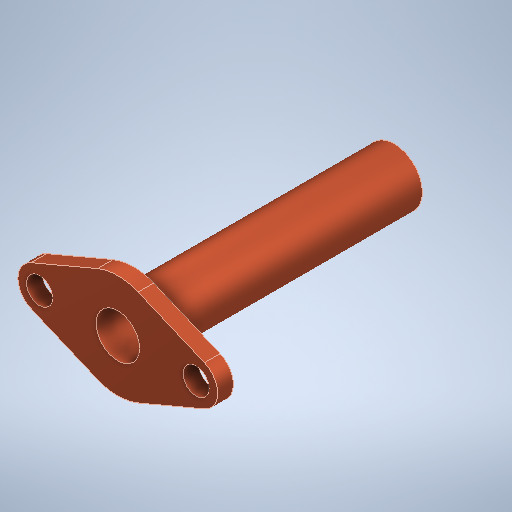
# Autodesk Inventor part: 36 - Inlet Outlet Steam Pipe
Saved by Autodesk Inventor 2025.2 (Build 292293000, 293)
## iProperties
Created: 2025-07-30
Part Number: 36 - Inlet Outlet Steam Pipe
Material: Copper
Document SubType Name: Modeling
Designer: bless
Density: 8.94 g/cm^3
Appearance: Copper - Satin
Author: bless
Autodesk Inventor part; units mm, degrees
ref_plane "YZ Plane" through (0, 0, 0) normal (1, 0, 0) x (0, 1, 0)
ref_plane "XZ Plane" through (0, 0, 0) normal (0, 1, 0) x (-1, 0, 0)
ref_plane "XY Plane" through (0, 0, 0) normal (0, 0, 1) x (1, 0, 0)
sketch "Sketch1" plane through (0, 0, 0) normal (0, 0, 1) x (1, 0, 0)
  circle A0 centre (0, 0) radius 2.5
  circle A1 centre (9, 0) radius 1.5
  circle A2 centre (-9, 0) radius 1.5
  circle A3 centre (-9, 0) radius 2.5
  circle A4 centre (9, 0) radius 2.5
  circle A5 centre (0, 0) radius 6
  line L0 (-9.9722, 2.3032) -> (-2.3333, 5.5277)
  line L1 (9.9722, 2.3032) -> (2.3333, 5.5277)
  line L2 (-9.9722, -2.3032) -> (-2.3333, -5.5277)
  line L3 (9.9722, -2.3032) -> (2.3333, -5.5277)
  dimension "d0" = 5
  dimension "d1" = 3
  dimension "d2" = 3
  dimension "d4" = 9
  dimension "d5" = 9
  dimension "d6" = 5
  dimension "d7" = 5
  dimension "d8" = 12
  constraints: 8 end point, 8 point on circle, 8 tangent, 6 centre point, 4 coincident, 2 horizontal alignment
  measures "d0" diameter of A0
  measures "d1" diameter of A1
  measures "d2" diameter of A2
  measures "d4" distance of A1.centre point (0, 0)
  measures "d5" distance of point (0, 0) A2.centre
  measures "d6" diameter of A3
  measures "d7" diameter of A4
  measures "d8" diameter of A5
extrude "Extrusion1" add sketch "Sketch1" against normal blind 1.8
sketch "Sketch2" plane through (0, 0, -1.8) normal (0, 0, -1) x (-1, 0, 0)
  circle A0 centre (0, 0) radius 2.5 projected
  circle A1 centre (0, 0) radius 3.25
  circle A2 centre (0, 0) radius 2.5
  dimension "d11" = 6.5
  dimension "d12" = 5
  constraints: 2 centre point, 2 coincident
  measures "d11" diameter of A1
  measures "d12" diameter of A2
extrude "Extrusion2" add sketch "Sketch2" along normal blind 30
body "Solid1"
